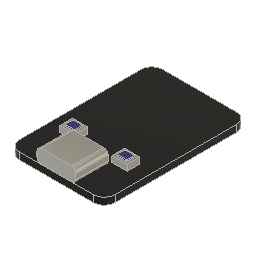
PLv3 Enclosure (Autodesk Fusion 360 archive; units mm, degrees)
design "Addon Module - USB"
Autodesk Fusion 360 part; units mm, degrees
sketch "Sketch1" plane through (0, 0, 0) normal (0, 0, 1) x (1, 0, 0) in component "USB_PCB"
  line L0 (8.5, 16.5) -> (-8.5, 16.5)
  line L1 (-11, 14) -> (-11, -14)
  line L2 (-8.5, -16.5) -> (8.5, -16.5)
  line L3 (11, -14) -> (11, 14)
  line L4 (11, 16.5) -> (-11, -16.5) construction
  line L5 (-11, 16.5) -> (11, -16.5) construction
  arc A0 (-8.5, 16.5) -> (-11, 14) centre (-8.5, 14) ccw
  arc A1 (11, 14) -> (8.5, 16.5) centre (8.5, 14) ccw
  arc A2 (8.5, -16.5) -> (11, -14) centre (8.5, -14) ccw
  arc A3 (-11, -14) -> (-8.5, -16.5) centre (-8.5, -14) ccw
  point P0 (0, -16.5)
  point P1 (-11, -16.5)
  point P2 (11, -16.5)
  dimension "d4" = 22
  dimension "d5" = 33
  dimension "d7" = 2.5
  constraint horizontal L0
  constraint perpendicular L0 L1
  constraint parallel L0 L2
  constraint parallel L1 L3
  constraint coincident L4 origin
  constraint coincident L5 origin
  constraint coincident L5.start L0
  constraint coincident L5.start L1
  constraint tangent L0 A0
  constraint tangent L1 A0
  constraint coincident L4.start L0
  constraint coincident L4.start L3
  constraint tangent L0 A1
  constraint tangent L3 A1
  constraint equal A0 A1
  constraint coincident P2 L2
  constraint coincident P2 L3
  constraint tangent L2 A2
  constraint tangent L3 A2
  constraint equal A0 A2
  constraint coincident P1 L1
  constraint coincident P1 L2
  constraint tangent L1 A3
  constraint tangent L2 A3
  constraint equal A0 A3
  constraint midpoint L2 P0
  constraint coincident P1 L4.end
  constraint coincident P2 L5.end
  measures "d4" distance of P1 P2
  measures "d5" distance of L5.start P1
  measures "d7" radius of A0
extrude "Extrude1" add sketch "Sketch1" along normal blind 1.6 makes body 1 in component "USB_PCB"
sketch "Sketch2" plane through (0, 0, 1.6) normal (0, 0, 1) x (-1, 0, 0) in component "USB_PCB"
  arc A0 (11, 14) -> (8.5, 16.5) centre (8.5, 14) ccw
  line L0 (8.5, 16.5) -> (-8.5, 16.5)
  arc A1 (-8.5, 16.5) -> (-11, 14) centre (-8.5, 14) ccw
  line L1 (-11, 14) -> (-11, -14)
  arc A2 (-11, -14) -> (-8.5, -16.5) centre (-8.5, -14) ccw
  line L2 (-8.5, -16.5) -> (8.5, -16.5)
  arc A3 (8.5, -16.5) -> (11, -14) centre (8.5, -14) ccw
  line L3 (11, -14) -> (11, 14)
  line L4 (-6, -16.5) -> (-6, 16.5) construction
  line L5 (6, -16.5) -> (6, 16.5) construction
  line L6 (11, 6.5) -> (-11, 6.5) construction
  line L7 (4.25, 5.05) -> (7.75, 5.05)
  line L8 (7.75, 5.05) -> (7.75, 7.95)
  line L9 (7.75, 7.95) -> (4.25, 7.95)
  line L10 (4.25, 7.95) -> (4.25, 5.05)
  line L11 (4.25, 5.05) -> (7.75, 7.95) construction
  line L12 (7.75, 5.05) -> (4.25, 7.95) construction
  line L13 (-7.75, 5.05) -> (-4.25, 5.05)
  line L14 (-4.25, 5.05) -> (-4.25, 7.95)
  line L15 (-4.25, 7.95) -> (-7.75, 7.95)
  line L16 (-7.75, 7.95) -> (-7.75, 5.05)
  line L17 (-7.75, 5.05) -> (-4.25, 7.95) construction
  line L18 (-4.25, 5.05) -> (-7.75, 7.95) construction
  line L19 (0, -16.5) -> (0, 16.5) construction
  line L20 (-11, 9.1) -> (11, 9.1) construction
  line L21 (11, 12.8) -> (-11, 12.8) construction
  line L22 (-4.5, 9.1) -> (4.5, 9.1)
  line L23 (4.5, 9.1) -> (4.5, 16.5)
  line L24 (4.5, 16.5) -> (-4.5, 16.5)
  line L25 (-4.5, 16.5) -> (-4.5, 9.1)
  line L26 (-4.5, 9.1) -> (4.5, 16.5) construction
  line L27 (4.5, 9.1) -> (-4.5, 16.5) construction
  point P0 (6, 6.5)
  point P1 (-6, 6.5)
  point P2 (0, 12.8)
  dimension "d12" = 10
  dimension "d13" = 5
  dimension "d14" = 5
  dimension "d18" = 3.5
  dimension "d19" = 2.9
  dimension "d20" = 3.5
  dimension "d21" = 2.9
  dimension "d36" = 7.4
  dimension "d37" = 3.7
  dimension "d38" = 9
  dimension "d39" = 7.4
  constraint coincident L2 L4.start
  constraint coincident L0 L4.end
  constraint perpendicular L0 L4
  constraint coincident L2 L5.start
  constraint coincident L0 L5.end
  constraint perpendicular L0 L5
  constraint coincident L3 L6.start
  constraint coincident L1 L6.end
  constraint perpendicular L1 L6
  constraint horizontal L7
  constraint perpendicular L7 L8
  constraint parallel L7 L9
  constraint parallel L8 L10
  constraint coincident L11 P0
  constraint coincident L12 P0
  constraint coincident L6 P0
  constraint coincident L5 P0
  constraint horizontal L13
  constraint perpendicular L13 L14
  constraint parallel L13 L15
  constraint parallel L14 L16
  constraint coincident L17 P1
  constraint coincident L18 P1
  constraint coincident L6 P1
  constraint coincident L4 P1
  constraint midpoint L2 L19.start
  constraint midpoint L0 L19.end
  constraint coincident L1 L20.start
  constraint coincident L3 L20.end
  constraint perpendicular L3 L20
  constraint coincident L3 L21.start
  constraint coincident L1 L21.end
  constraint perpendicular L1 L21
  constraint horizontal L22
  constraint perpendicular L22 L23
  constraint parallel L22 L24
  constraint parallel L23 L25
  constraint coincident L26 P2
  constraint coincident L27 P2
  constraint midpoint L21 P2
  measures "d12" distance of L0 L6
  measures "d13" distance of L3 L5
  measures "d14" distance of L1 L4
  measures "d18" distance of L8.end L9.end
  measures "d19" distance of L7.end L8.end
  measures "d20" distance of L14.end L15.end
  measures "d21" distance of L13.end L14.end
  measures "d36" distance of L0 L20
  measures "d37" distance of L0 L21
  measures "d38" distance of L23.end L24.end
  measures "d39" distance of L22.end L23.end
extrude "Extrude2" add sketch "Sketch2" along normal blind 1.4 separate body contours L7 L8 L9 L10 | L13 L14 L15 L16 makes body 2 at (-5.4167, -6.0167, 1.6) makes body 3 at (6.5833, -6.0167, 1.6) in component "USB_PCB"
sketch "Sketch3" plane through (0, 0, 3) normal (0, 0, 1) x (-1, 0, 0) in component "USB_PCB"
  line L0 (4.25, 7.95) -> (4.25, 5.05)
  line L1 (4.25, 5.05) -> (7.75, 5.05)
  line L2 (7.75, 5.05) -> (7.75, 7.95)
  line L3 (7.75, 7.95) -> (4.25, 7.95)
  line L4 (6, 5.05) -> (6, 7.95) construction
  line L5 (-7.75, 7.95) -> (-7.75, 5.05) construction
  line L6 (7.75, 6.5) -> (-7.75, 6.5) construction
  line L7 (-7.75, 5.05) -> (-4.25, 5.05) construction
  line L8 (-4.25, 7.95) -> (-7.75, 7.95) construction
  line L9 (-6, 5.05) -> (-6, 7.95) construction
  line L10 (4.9, 5.6) -> (7.1, 5.6)
  line L11 (7.1, 5.6) -> (7.1, 7.4)
  line L12 (7.1, 7.4) -> (4.9, 7.4)
  line L13 (4.9, 7.4) -> (4.9, 5.6)
  line L14 (4.9, 5.6) -> (7.1, 7.4) construction
  line L15 (7.1, 5.6) -> (4.9, 7.4) construction
  line L16 (-7.1, 5.6) -> (-4.9, 5.6)
  line L17 (-4.9, 5.6) -> (-4.9, 7.4)
  line L18 (-4.9, 7.4) -> (-7.1, 7.4)
  line L19 (-7.1, 7.4) -> (-7.1, 5.6)
  line L20 (-7.1, 5.6) -> (-4.9, 7.4) construction
  line L21 (-4.9, 5.6) -> (-7.1, 7.4) construction
  point P0 (6, 6.5)
  point P1 (-6, 6.5)
  dimension "d27" = 2.2
  dimension "d28" = 1.8
  dimension "d29" = 2.2
  dimension "d30" = 1.8
  constraint midpoint L1 L4.start
  constraint midpoint L3 L4.end
  constraint midpoint L2 L6.start
  constraint midpoint L5 L6.end
  constraint midpoint L7 L9.start
  constraint midpoint L8 L9.end
  constraint horizontal L10
  constraint perpendicular L10 L11
  constraint parallel L10 L12
  constraint parallel L11 L13
  constraint coincident L14 P0
  constraint coincident L15 P0
  constraint midpoint L4 P0
  constraint horizontal L16
  constraint perpendicular L16 L17
  constraint parallel L16 L18
  constraint parallel L17 L19
  constraint coincident L20 P1
  constraint coincident L21 P1
  constraint midpoint L9 P1
  measures "d27" distance of L11.end L12.end
  measures "d28" distance of L10.end L11.end
  measures "d29" distance of L17.end L18.end
  measures "d30" distance of L16.end L17.end
extrude "Extrude3" add sketch "Sketch3" along normal blind 0.3 separate body contours L10 L11 L12 L13 | L16 L17 L18 L19 makes body 4 at (-6.3667, -6.2, 3) makes body 5 at (5.6333, -6.2, 3) in component "USB_PCB"
extrude "Extrude4" add sketch "Sketch2" along normal blind 3.2 separate body contours L0 L22 L23 L24 L25 makes body 6 in component "USB_PCB"
fillet "Fillet1" radius 1 4 edges at (-4.5, -12.8, 1.6) (-4.5, -12.8, 4.8) (4.5, -12.8, 4.8) (4.5, -12.8, 1.6) on bodies 6 in component "USB_PCB"
component "USB_PCB" placed x (1, 0, 0) y (0, 1, 0) z (0, 0, 1) at (0, 0, 0)
equation "Board_Width = 22 mm"
equation "Board_Height = 33 mm"
equation "PCB_Thickness = 1.6 mm"
equation "d4 = Board_Width"
equation "d5 = Board_Height"
equation "Board_Fillet_Radius = 2.5 mm"
equation "d7 = Board_Fillet_Radius"
equation "d8 = PCB_Thickness"
equation "Button_Up_Offset = 10 mm"
equation "Button_In_Offset = 5 mm"
equation "d12 = Button_Up_Offset"
equation "d13 = Button_In_Offset"
equation "d14 = Button_In_Offset"
equation "Button_Width = 3.5 mm"
equation "Button_Height = 2.9 mm"
equation "Button_Depth = 1.4 mm"
equation "d18 = Button_Width"
equation "d19 = Button_Height"
equation "d20 = Button_Width"
equation "d21 = Button_Height"
equation "d22 = Button_Depth"
equation "Button_Nipple_Width = 2.2 mm"
equation "Button_Nipple_Height = 1.8 mm"
equation "Button_Nipple_Depth = 0.3 mm"
equation "d27 = Button_Nipple_Width"
equation "d28 = Button_Nipple_Height"
equation "d29 = Button_Nipple_Width"
equation "d30 = Button_Nipple_Height"
equation "d31 = Button_Nipple_Depth"
equation "USB_Width = 9 mm"
equation "USB_Height = 7.4 mm"
equation "USB_Depth = 3.2 mm"
equation "d36 = USB_Height"
equation "d37 = USB_Height / 2"
equation "d38 = USB_Width"
equation "d39 = USB_Height"
equation "d40 = USB_Depth"
equation "USB_Radius = 1 mm"
equation "d44 = USB_Radius"
